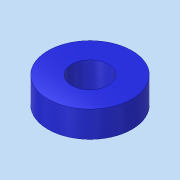
# Autodesk Inventor part: Unterlagscheibe
Saved by Autodesk Inventor 2018 (Build 220112000, 112)
## iProperties
Created: 2020-10-03
Part Number: Unterlagscheibe
Material: Generisch
Document SubType Name: Modeling
Designer: marce
Density: 1 g/cm^3
Appearance: Blau - Wandfarbe - glänzend
Author: marce
Autodesk Inventor part; units mm, degrees
ref_plane "YZ Plane" through (0, 0, 0) normal (1, 0, 0) x (0, 1, 0)
ref_plane "XZ Plane" through (0, 0, 0) normal (0, 1, 0) x (-1, 0, 0)
ref_plane "XY Plane" through (0, 0, 0) normal (0, 0, 1) x (1, 0, 0)
sketch "Skizze1" plane through (0, 0, 0) normal (0, 0, 1) x (1, 0, 0)
  circle A0 centre (0, 0) radius 1.75
  circle A1 centre (0, 0) radius 4
  dimension "d0" = 3.5
  dimension "d1" = 8
  constraints: 2 centre point, 2 coincident
  measures "d0" diameter of A0
  measures "d1" diameter of A1
extrude "Extrusion1" add sketch "Skizze1" along normal blind 2.5
